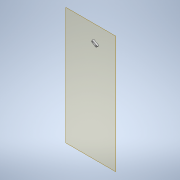
# Autodesk Inventor part: backcover_clamp_mini
Saved by Autodesk Inventor 2020 (Build 240168000, 168)
## iProperties
Created: 2019-07-29
Part Number: backcover_clamp_mini
Material: Generic
Document SubType Name: Modeling
Designer: erwin
Density: 1 g/cm^3
Appearance: Default
Author: erwin
Autodesk Inventor part; units mm, degrees
ref_plane "YZ Plane" through (0, 0, 0) normal (1, 0, 0) x (0, 1, 0)
ref_plane "XZ Plane" through (0, 0, 0) normal (0, 1, 0) x (-1, 0, 0)
ref_plane "XY Plane" through (0, 0, 0) normal (0, 0, 1) x (1, 0, 0)
ref_plane "Work Plane1" through (0, 0, 0) normal (0, 0, 1) x (1, 0, 0)
sketch "Sketch1" plane through (0, 0, 0) normal (0, 0, 1) x (1, 0, 0)
  line L0 (39.878985, 283.001047) -> (46.807188, 279.001047)
  line L1 (118.687297, 237.501047) -> (-32.001123, 324.501047)
  line L2 (118.687297, 237.501047) -> (112.687297, 227.108743)
  line L3 (-38.001123, 314.108743) -> (112.687297, 227.108743)
  line L4 (-32.001123, 324.501047) -> (-38.001123, 314.108743)
  line L5 (40.807188, 268.608743) -> (46.807188, 279.001047)
  line L6 (33.878985, 272.608743) -> (39.878985, 283.001047)
  line L7 (40.807188, 268.608743) -> (33.878985, 272.608743)
  circle A0 centre (68.259454, 214.654052) radius 27.5 construction
  line L8 (52.931544, 261.608743) -> (21.754629, 279.608743)
  line L9 (21.754629, 279.608743) -> (15.754629, 269.216438)
  line L10 (15.754629, 269.216438) -> (46.931544, 251.216438)
  line L11 (46.931544, 251.216438) -> (52.931544, 261.608743)
  point P0 (0, 0)
  dimension "d0" = 55
  dimension "d1" = 12
  dimension "d2" = 14
  dimension "d3" = 14
  constraints: 12 end point, 2 parallel, 2 point on line, 1 centre point, 1 coincident, 1 perpendicular, 4 other
  measures "d0" diameter of A0
  measures "d1" distance of L9.end L8.end
  measures "d2" distance between parallel lines of L9 L6
  measures "d3" distance between parallel lines of L5 L11
sketch "Sketch1 outline for Extrusion1" plane through (0, 0, 0) normal (0, 0, 1) x (1, 0, 0)
  line L0 (15.754629, 269.216438) -> (46.931544, 251.216438)
  line L1 (21.754629, 279.608743) -> (15.754629, 269.216438)
  line L2 (52.931544, 261.608743) -> (21.754629, 279.608743)
  line L3 (46.931544, 251.216438) -> (52.931544, 261.608743)
extrude "Extrusion1" add sketch "Sketch1 outline for Extrusion1" along normal blind 10
fillet "Fillet1" radius 6 2 edges at (15.7546, 269.2164, 5) (46.9315, 251.2164, 5)
sketch "Sketch2" plane through (0, 0, 10) normal (0, 0, 1) x (1, 0, 0)
  arc A0 (18.754629, 274.41259) -> (20.950782, 266.216438) centre (23.950782, 271.41259) ccw
  arc A1 (41.735391, 254.216438) -> (49.931544, 256.41259) centre (44.735391, 259.41259) ccw
  point P0 (0, 0)
  constraints: 2 coincident
hole "Hole1" at (23.950782, 271.41259, 10) at (44.735391, 259.41259, 10) direction (0, 0, -1) diameter 3.5 end through all countersink diameter 8 countersink angle 90
sketch "Sketch3" plane through (0, 0, 10) normal (0, 0, 1) x (1, 0, 0)
  line L0 (52.931544, 261.608743) -> (21.754629, 279.608743)
  line L1 (42.539239, 267.608743) -> (32.146934, 273.608743)
  line L2 (32.146934, 273.608743) -> (26.146934, 263.216438)
  line L3 (26.146934, 263.216438) -> (36.539239, 257.216438)
  line L4 (36.539239, 257.216438) -> (42.539239, 267.608743)
  line L5 (21.754629, 279.608743) -> (18.754629, 274.41259)
  line L6 (49.931544, 256.41259) -> (52.931544, 261.608743)
  point P0 (0, 0)
  dimension "d14" = 12
  dimension "d15" = 12
  dimension "d16" = 12
  constraints: 8 end point, 2 parallel, 2 point on line, 1 perpendicular
  measures "d14" distance between parallel lines of L4 L2
  measures "d15" distance between parallel lines of L5 L2
  measures "d16" distance between parallel lines of L6 L4
sketch "Sketch3 outline for Extrusion2" plane through (0, 0, 10) normal (0, 0, 1) x (1, 0, 0)
  line L0 (26.146934, 263.216438) -> (36.539239, 257.216438)
  line L1 (32.146934, 273.608743) -> (26.146934, 263.216438)
  line L2 (42.539239, 267.608743) -> (32.146934, 273.608743)
  line L3 (36.539239, 257.216438) -> (42.539239, 267.608743)
extrude "Extrusion2" add sketch "Sketch3 outline for Extrusion2" along normal blind 47
sketch "Sketch4" plane through (21.754629, 279.608743, 10) normal (0.5, 0.8660254, 0) x (0.8660254, -0.5, 0)
  circle A0 centre (18, -41) radius 4 projected
  point P0 (120.96431, 10)
sketch "Sketch4 outline for Extrusion3" plane through (21.754629, 279.608743, 10) normal (0.5, 0.8660254, 0) x (0.8660254, -0.5, 0)
  circle A0 centre (18, -41) radius 4
extrude "Extrusion3" cut sketch "Sketch4 outline for Extrusion3" against normal through all
fillet "Fillet2" radius 6 2 edges at (39.5392, 262.4126, 57) (29.1469, 268.4126, 57)
fillet "Fillet3" radius 1 2 edges at (29.1469, 268.4126, 10) (39.5392, 262.4126, 10)
draft "FaceDraft1" angle 2 pull direction (0, 0, 1) faces at (37.48227, 270.528385, 23.009722) fixed edges at (37.343087, 270.608743, 0)
sketch "Sketch6" plane through (49.931544, 256.41259, 10) normal (0.8660254, -0.5, 0) x (0, 0, -1)
  line L0 (0, 0) -> (0, -6)
  line L1 (0, -6) -> (10, -6)
  line L2 (10, -6) -> (10, 0)
  line L3 (10, 0) -> (0, 0)
  line L4 (10, 0) -> (0, 0)
  line L5 (10, 0) -> (10, 6)
  line L6 (10, 6) -> (0, 5.650792)
  line L7 (0, 0) -> (0, 5.650792)
  line L8 (-1, -6) -> (0, -6)
  line L9 (0, -6) -> (-53.172101, -6)
  line L10 (-53.172101, -6) -> (-53.172101, 15.66156)
  line L11 (-53.172101, 15.66156) -> (0, 15.66156)
  line L12 (0, 15.66156) -> (0, -6)
  point P0 (10, -247.025589)
  point P1 (0, 5.650792)
  constraints: 8 end point, 2 parallel, 1 horizontal, 1 perpendicular
sketch "Sketch6 outline for Extrusion4" plane through (49.931544, 256.41259, 10) normal (0.8660254, -0.5, 0) x (0, 0, -1)
  line L0 (0, 15.66156) -> (-53.172101, 15.66156)
  line L1 (0, 5.650792) -> (0, 15.66156)
  line L2 (0, 0) -> (0, 5.650792)
  line L3 (0, -6) -> (0, 0)
  line L4 (-1, -6) -> (0, -6)
  line L5 (-53.172101, -6) -> (-1, -6)
  line L6 (-53.172101, 15.66156) -> (-53.172101, -6)
extrude "Extrusion4" cut sketch "Sketch6 outline for Extrusion4" against normal through all
equation "\"d2\" = d3"
equation "\"d15\" = d16"
body "Solid1"
